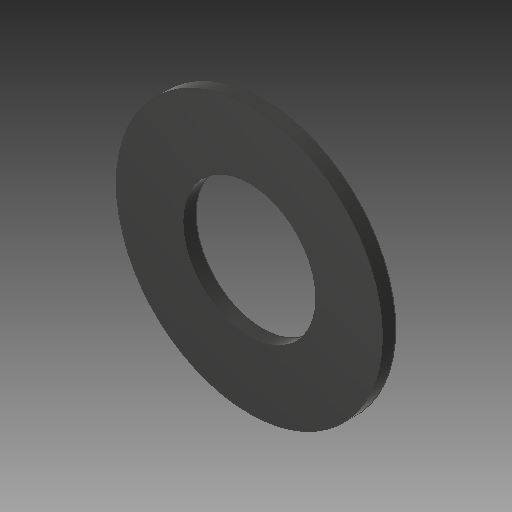
# Autodesk Inventor part: ワッシャ10-20  1
Saved by Autodesk Inventor 2017.3 (Build 213256000, 256)
## iProperties
Part Number: ワッシャ10-20  1
Material: アセタール樹脂、黒
Document SubType Name: Modeling
Designer: 原知也
Density: 1.425 g/cm^3
Appearance: 滑らか - 黒
Mass: 0.335758 g
Surface Area: 5.65487 cm^2
Volume: 0.235619 cm^3
Author: 原知也
Autodesk Inventor part; units mm, degrees
ref_plane "YZ Plane" through (0, 0, 0) normal (1, 0, 0) x (0, 1, 0)
ref_plane "XZ Plane" through (0, 0, 0) normal (0, 1, 0) x (-1, 0, 0)
ref_plane "XY Plane" through (0, 0, 0) normal (0, 0, 1) x (1, 0, 0)
sketch "スケッチ1" plane through (0, 0, 0) normal (0, 0, 1) x (1, 0, 0)
  circle A0 centre (0, 0) radius 5
  circle A1 centre (0, 0) radius 10
  dimension "d0" = 10
  dimension "d1" = 20
  constraints: 2 centre point, 2 coincident
  measures "d0" diameter of A0
  measures "d1" diameter of A1
extrude "押し出し1" add sketch "スケッチ1" along normal blind 1
